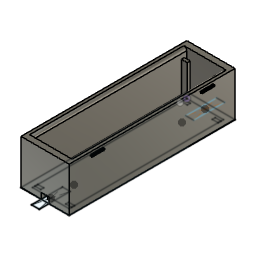
single battery holder and lid 5 (Autodesk Fusion 360 design; units mm, degrees)
Autodesk Fusion 360 part; units mm, degrees
note: some values were not read from the file. Set by a fixed rule: which face or edge a step refers to.
sketch "Sketch1" plane through (0, 0, 0) normal (0, 0, 1) x (1, 0, 0)
  line L0 (0, 0) -> (19, 0)
  line L1 (19, 0) -> (19, -80)
  line L2 (19, -80) -> (0, -80)
  line L3 (0, -80) -> (0, 0)
  line L4 (22, 3) -> (22, -83)
  line L5 (22, -83) -> (-3, -83)
  line L6 (-3, -83) -> (-3, 3)
  line L7 (-3, 3) -> (22, 3)
  line L8 (0, -3.5) -> (0, -1.25)
  line L9 (19, -1.25) -> (16, -1.25)
  line L10 (16, -1.25) -> (16, -2.75)
  line L11 (16, -2.75) -> (19, -2.75)
  line L12 (19, -2.75) -> (19, -1.25)
  line L13 (0, -77.25) -> (3, -77.25)
  line L14 (3, -77.25) -> (3, -78.75)
  line L15 (3, -78.75) -> (0, -78.75)
  line L16 (0, -78.75) -> (0, -77.25)
  line L17 (19, -77.25) -> (16, -77.25)
  line L18 (16, -77.25) -> (16, -78.75)
  line L19 (16, -78.75) -> (19, -78.75)
  line L20 (19, -78.75) -> (19, -77.25)
  line L21 (0, -1.25) -> (3, -1.25)
  line L22 (3, -1.25) -> (3, -2.75)
  line L23 (3, -2.75) -> (0, -2.75)
  line L24 (0, -2.75) -> (0, -1.25)
  line L25 (11.5, -8) -> (7.5, -8)
  line L26 (7.5, -8) -> (7.5, 8)
  line L27 (7.5, 8) -> (11.5, 8)
  line L28 (11.5, 8) -> (11.5, -8)
  line L29 (11.5, -8) -> (7.5, 8) construction
  line L30 (7.5, -8) -> (11.5, 8) construction
  line L31 (11.5, -88) -> (7.5, -88)
  line L32 (7.5, -88) -> (7.5, -72)
  line L33 (7.5, -72) -> (11.5, -72)
  line L34 (11.5, -72) -> (11.5, -88)
  line L35 (11.5, -88) -> (7.5, -72) construction
  line L36 (7.5, -88) -> (11.5, -72) construction
  point P0 (9.5, 0)
  point P1 (9.5, -80)
  point P2 (9.5, -12)
  point P3 (9.5, -68)
  dimension "d1" = 80
  dimension "d2" = 19
  dimension "d3" = -3
  dimension "d5" = 3
  dimension "d6" = 1.5
  dimension "d7" = 3
  dimension "d8" = 1.5
  dimension "d9" = 3
  dimension "d10" = 1.5
  dimension "d11" = 1.5
  dimension "d12" = 3
  dimension "d13" = 1.25
  dimension "d14" = 1.25
  dimension "d15" = 1.25
  dimension "d16" = 1.25
  dimension "d19" = 12
  dimension "d20" = 12
  dimension "d28" = 16
  dimension "d29" = 16
  dimension "d30" = 4
  constraint horizontal L0
  constraint vertical L1
  constraint horizontal L2
  constraint vertical L3
  constraint coincident L0.start L3.end
  constraint vertical L8
  constraint coincident L3 L8.end
  constraint horizontal L9
  constraint vertical L10
  constraint horizontal L11
  constraint vertical L12
  constraint coincident L1 L9.start
  constraint horizontal L13
  constraint vertical L14
  constraint horizontal L15
  constraint vertical L16
  constraint coincident L3 L13.start
  constraint horizontal L17
  constraint vertical L18
  constraint horizontal L19
  constraint vertical L20
  constraint coincident L1 L17.start
  constraint horizontal L21
  constraint vertical L22
  constraint horizontal L23
  constraint vertical L24
  constraint perpendicular L25 L26
  constraint parallel L25 L27
  constraint parallel L26 L28
  constraint horizontal L25
  constraint coincident L29 P0
  constraint coincident L30 P0
  constraint midpoint L0 P0
  constraint perpendicular L31 L32
  constraint parallel L31 L33
  constraint parallel L32 L34
  constraint horizontal L31
  constraint coincident L35 P1
  constraint coincident L36 P1
  constraint midpoint L2 P1
  constraint vertical P1 P3
  constraint vertical P0 P2
  measures "d1" distance of L0.start L2.end
  measures "d2" distance of L0.start L0.end
  measures "d5" distance of L9.start L9.end
  measures "d6" distance of L9.start L11.end
  measures "d7" distance of L13.start L13.end
  measures "d8" distance of L13.start L15.end
  measures "d9" distance of L17.start L17.end
  measures "d10" distance of L17.start L19.end
  measures "d11" distance of L8.end L23.end
  measures "d12" distance of L8.end L21.end
  measures "d13" distance of L0 L21.end
  measures "d14" distance of L0 L9.end
  measures "d15" distance of L2 L14.end
  measures "d16" distance of L2 L18.end
  measures "d19" distance of L0 P2
  measures "d20" distance of L2 P3
  measures "d28" distance of L25.end L26.end
  measures "d29" distance of L31.end L32.end
  measures "d30" distance of L32.end L33.end
extrude "Extrude1" add sketch "Sketch1" along normal blind 3 contours L0 L1 L2 L3 L8 L9 L10 L11 L13 L14 L15 L17 L18 L19 L21 L22 L23 L25 L26 L28 L32 L33 L34 makes body 1
extrude "Extrude1'" add sketch "Sketch1" along normal blind 23 separate body contours L0 L2 L3 L5 L6 L7 L8 L16 L24 L26 L32 | L0 L7 L26 L28 | L0 L1 L2 L4 L5 L7 L12 L20 L28 L34 | L2 L5 L32 L34 makes body 2 in component "single battery holder"
sketch "Sketch1 (2)" plane through (0, 0, 0) normal (0, -1, 0) x (1, 0, 0) in component "single battery holder"
  line L0 (0, 0) -> (19, 0)
  line L1 (19, 0) -> (19, 23)
  line L2 (19, 23) -> (0, 23)
  line L3 (0, 23) -> (0, 0)
  line L4 (-3, 0) -> (22.0074, 23) construction
  line L5 (22.0074, 23) -> (-3, 23) construction
  line L6 (-3, 23) -> (22, 0) construction
  circle A0 centre (9.5037, 11.5) radius 9.5
  dimension "d23" = 19
  constraint perpendicular L3 L5
  constraint midpoint L4 A0.centre
  measures "d23" diameter of A0
extrude "Extrude2" cut sketch "Sketch1 (2)" along normal blind 80 contours L1 A0 | L1 A0 bodies 2 in component "single battery holder"
extrude "Extrude3" add sketch "Sketch1" along normal blind 19 contours L3 L8 L21 L22 L23 L24 | L1 L9 L10 L11 L12 | L3 L13 L14 L15 L16 | L1 L17 L18 L19 L20 bodies 2 in component "single battery holder"
fillet "Fillet1" radius 1.5 2 edges at (0, -40, 23) (19, -40, 23) on bodies 2 in component "single battery holder"
hole "Hole1" at (9.5, -17, 3) direction (0, 0, -1) diameter 3 depth 4 tip angle 180 countersink diameter 4.5 countersink angle 90 bodies 1
hole "Hole2" at (9.5, -63, 3) direction (0, 0, -1) diameter 3 depth 4 tip angle 118 countersink diameter 4.5 countersink angle 90 bodies 1
extrude "Extrude6" cut sketch "Sketch1" along normal blind 3 contours L0 L7 L26 L28 | L2 L5 L32 L34 bodies 2 in component "single battery holder"
sketch "Sketch2" plane through (-3, 0, 0) normal (-1, 0, 0) x (0, -1, 0) in component "single battery holder"
  line L0 (-3, 0) -> (83, 0)
  line L1 (83, 0) -> (83, 23)
  line L2 (83, 23) -> (-3, 23)
  line L3 (-3, 23) -> (-3, 0)
  line L4 (-3, 23) -> (83, 0) construction
  line L5 (-3, 0) -> (83, 23) construction
  line L6 (35, 13) -> (45, 10) construction
  line L7 (45, 13) -> (35, 10) construction
  point P0 (40, 11.5)
  constraint coincident L2.end L3.start
  constraint coincident L0.end L1.start
  constraint coincident L0.start L3.end
  constraint coincident L1.end L2.start
  constraint coincident L6 P0
  constraint coincident L7 P0
  constraint midpoint L5 P0
combine "Combine1" operation add target body 2 tool bodies 1 in component "single battery holder"
ref_plane "WorkPlane1" through (9.5, -83.25, 11.5) normal (0, -1, 0) x (1, 0, 0) in component "Lid4"
sketch "Sketch1 (3)" plane through (9.5, -83.25, 11.5) normal (0, -1, 0) x (1, 0, 0) in component "Lid4"
  line L0 (2, -8.5) -> (2, -11.5)
  line L1 (2, -11.5) -> (12.5, -11.5)
  line L2 (12.5, -11.5) -> (12.5, 11.5)
  line L3 (12.5, 11.5) -> (-12.5, 11.5)
  line L4 (-12.5, 11.5) -> (-12.5, -11.5)
  line L5 (-12.5, -11.5) -> (-2, -11.5)
  line L6 (-2, -11.5) -> (-2, -8.5)
  line L7 (-2, -8.5) -> (2, -8.5)
  line L8 (-13, 7.9743) -> (-15, 7.9743)
  line L9 (-15, 7.9743) -> (-15, 13.501)
  line L10 (-15, 13.501) -> (15, 13.501)
  line L11 (15, 13.501) -> (15, 7.9743)
  line L12 (15, 7.9743) -> (13, 7.9743)
  line L13 (13, 7.9743) -> (13, 11.501)
  line L14 (13, 11.501) -> (-13, 11.501)
  line L15 (-13, 11.501) -> (-13, 7.9743)
  line L16 (0, 11.5) -> (0, 21.153) construction
  line L17 (-12.5, -11.5) -> (-12.5, 11.5)
  line L18 (12.5074, 11.5) -> (-12.5, 11.5)
  dimension "d157" = 0.5
  dimension "d158" = 2
  dimension "d159" = 0.001
  dimension "d160" = 2
  constraint perpendicular L4 L8
  constraint perpendicular L8 L9
  constraint perpendicular L4 L10
  constraint perpendicular L10 L11
  constraint perpendicular L11 L12
  constraint perpendicular L12 L13
  constraint perpendicular L11 L14
  constraint perpendicular L8 L15
  constraint midpoint L3 L16.start
  constraint perpendicular L3 L16
  constraint symmetric L8.start L12.end L16
  constraint symmetric L8.end L11.end L16
  measures "d157" distance of L8.start L17
  measures "d158" distance of L8.start L8.end
  measures "d159" distance of L14 L18
  measures "d160" distance of L10 L14
extrude "Extrude1''" add sketch "Sketch1 (3)" along normal blind 0.35 and the other way blind 86.75 separate body contours L3 L8 L9 L10 L11 L12 L13 L14 L15 L18 makes body 3 in component "Lid4"
sketch "Sketch2 (2)" plane through (24.5, 0, 0) normal (1, 0, 0) x (0, 1, 0) in component "Lid4"
  line L0 (3.5, 25.001) -> (-83.6, 25.001)
  line L1 (-83.6, 25.001) -> (-83.6, 19.4743)
  line L2 (-83.6, 19.4743) -> (3.5, 19.4743)
  line L3 (3.5, 19.4743) -> (3.5, 25.001)
  line L4 (-83, 0) -> (3, 0)
  line L5 (3, 0) -> (3, 23)
  line L6 (3, 23) -> (-83, 23)
  line L7 (-83, 23) -> (-83, 0)
  line L8 (-83.6, 23) -> (3.5, 23) construction
  line L9 (-83.6, 23) -> (3.5, 23) construction
  line L10 (3.5, 23) -> (3.5, 19.4743) construction
  line L11 (3.5, 19.4743) -> (-83.6, 19.4743) construction
  line L12 (-83.6, 19.4743) -> (-83.6, 23) construction
  line L13 (-71.6, 20.4871) -> (-65.6, 20.4871)
  arc A0 (-65.6, 20.4871) -> (-65.6, 21.9871) centre (-65.6, 21.2371) ccw
  line L14 (-65.6, 21.9871) -> (-71.6, 21.9871)
  arc A1 (-71.6, 21.9871) -> (-71.6, 20.4871) centre (-71.6, 21.2371) ccw
  line L15 (-71.6, 21.2371) -> (-65.6, 21.2371) construction
  line L16 (-43.05, 20.4871) -> (-37.05, 20.4871)
  line L17 (-43.05, 21.2371) -> (-37.05, 21.2371) construction
  arc A2 (-37.05, 20.4871) -> (-37.05, 21.9871) centre (-37.05, 21.2371) ccw
  line L18 (-37.05, 21.9871) -> (-43.05, 21.9871)
  arc A3 (-43.05, 21.9871) -> (-43.05, 20.4871) centre (-43.05, 21.2371) ccw
  line L19 (-8.5, 21.9871) -> (-14.5, 21.9871)
  line L20 (-14.5, 20.4871) -> (-8.5, 20.4871)
  arc A4 (-14.5, 21.9871) -> (-14.5, 20.4871) centre (-14.5, 21.2371) ccw
  arc A5 (-8.5, 20.4871) -> (-8.5, 21.9871) centre (-8.5, 21.2371) ccw
  line L21 (-14.5, 21.2371) -> (-8.5, 21.2371) construction
  point P0 (-68.6, 21.2371)
  point P1 (-40.05, 21.2371)
  point P2 (-11.5, 21.2371)
  point P3 (-68.6, 21.2371)
  dimension "d165" = 3.5257
  dimension "d166" = 1.7629
  dimension "d168" = 15
  dimension "d169" = 15
  dimension "d170" = 43.55
  dimension "d171" = 3
  dimension "d172" = 1.5
  dimension "d173" = 1.5
  dimension "d174" = 1.5
  constraint coincident L1 L8.start
  constraint coincident L3 L8.end
  constraint perpendicular L5 L8
  constraint horizontal L9
  constraint vertical L10
  constraint horizontal L11
  constraint vertical L12
  constraint coincident L2.end L3.start
  constraint horizontal P3 P1
  constraint horizontal P1 P2
  constraint tangent L13 A0
  constraint tangent A0 L14
  constraint parallel L13 L14
  constraint tangent L14 A1
  constraint tangent L13 A1
  constraint parallel L8 L15
  constraint coincident P3 P0
  constraint midpoint L15 P3
  constraint tangent L16 A2
  constraint tangent A2 L18
  constraint parallel L16 L18
  constraint tangent L18 A3
  constraint tangent L16 A3
  constraint tangent L20 A5
  constraint tangent L19 A5
  constraint parallel L19 L20
  constraint tangent L19 A4
  constraint tangent L20 A4
  measures "d165" distance of L1.end L8.start
  measures "d166" distance of L8 P3
  measures "d168" distance of L12 P3
  measures "d169" distance of L3 P2
  measures "d170" distance of L10 P1
  measures "d171" distance of A0.centre P3
  measures "d172" diameter of A0
  measures "d173" diameter of A2
  measures "d174" diameter of A5
extrude "Extrude2'" cut sketch "Sketch2 (2)" along normal blind -3 and the other way blind 1 contours L13 A0 L14 A1 | L19 L20 A4 A5 bodies 3 in component "Lid4"
sketch "Sketch6" plane through (22, 0, 0) normal (1, 0, 0) x (0, 1, 0) in component "single battery holder"
  line L0 (-83, 0) -> (3, 0)
  line L1 (3, 0) -> (3, 23)
  line L2 (3, 23) -> (-83, 23)
  line L3 (-83, 23) -> (-83, 0)
  arc A0 (-8.5, 20.4871) -> (-8.5, 21.9871) centre (-8.5, 21.2371) ccw construction
  line L4 (-8.5, 20.4871) -> (-14.5, 20.4871) construction
  arc A1 (-14.5, 21.9871) -> (-14.5, 20.4871) centre (-14.5, 21.2371) ccw construction
  line L5 (-14.5, 21.9871) -> (-8.5, 21.9871) construction
  arc A2 (-71.6, 21.9871) -> (-71.6, 20.4871) centre (-71.6, 21.2371) ccw construction
  line L6 (-71.6, 21.9871) -> (-65.6, 21.9871) construction
  arc A3 (-65.6, 20.4871) -> (-65.6, 21.9871) centre (-65.6, 21.2371) ccw construction
  line L7 (-65.6, 20.4871) -> (-71.6, 20.4871) construction
  line L8 (-71.6, 21.2371) -> (-65.6, 21.2371) construction
  line L9 (-71.6, 20.6871) -> (-65.6, 20.6871)
  arc A4 (-65.6, 20.6871) -> (-65.6, 21.7871) centre (-65.6, 21.2371) ccw
  line L10 (-65.6, 21.7871) -> (-71.6, 21.7871)
  arc A5 (-71.6, 21.7871) -> (-71.6, 20.6871) centre (-71.6, 21.2371) ccw
  line L11 (-71.6, 21.2371) -> (-65.6, 21.2371) construction
  line L12 (-8.5, 21.2371) -> (-14.5, 21.2371) construction
  line L13 (-14.5, 20.6871) -> (-8.5, 20.6871)
  arc A6 (-8.5, 20.6871) -> (-8.5, 21.7871) centre (-8.5, 21.2371) ccw
  line L14 (-8.5, 21.7871) -> (-14.5, 21.7871)
  arc A7 (-14.5, 21.7871) -> (-14.5, 20.6871) centre (-14.5, 21.2371) ccw
  line L15 (-14.5, 21.2371) -> (-8.5, 21.2371) construction
  point P0 (-68.6, 21.2371)
  point P1 (-11.5, 21.2371)
  dimension "d179" = 1.1
  dimension "d180" = 1.1
  constraint coincident A2.centre L8.start
  constraint coincident A3.centre L8.end
  constraint tangent L9 A4
  constraint tangent A4 L10
  constraint parallel L9 L10
  constraint tangent L10 A5
  constraint tangent L9 A5
  constraint parallel L8 L11
  constraint midpoint L8 P0
  constraint midpoint L11 P0
  constraint coincident A0.centre L12.start
  constraint coincident A1.centre L12.end
  constraint tangent L13 A6
  constraint tangent A6 L14
  constraint parallel L13 L14
  constraint tangent L14 A7
  constraint tangent L13 A7
  constraint parallel L12 L15
  constraint midpoint L12 P1
  constraint midpoint L15 P1
  measures "d179" diameter of A4
  measures "d180" diameter of A6
extrude "Extrude11" add sketch "Sketch6" along normal blind 0.75 contours L9 A4 L10 A5 | L13 A6 L14 A7 bodies 2 in component "single battery holder"
fillet "Fillet5" radius 0.25 2 faces at (22.75, -10.5, 21.0538) (22.75, -67.6, 21.0538) on bodies 2 in component "single battery holder"
sketch "Sketch3" plane through (-5.5, 0, 0) normal (-1, 0, 0) x (0, -1, 0) in component "Lid4"
  line L0 (-3.5, 19.4743) -> (83.6, 19.4743)
  line L1 (83.6, 19.4743) -> (83.6, 25.001)
  line L2 (83.6, 25.001) -> (-3.5, 25.001)
  line L3 (-3.5, 25.001) -> (-3.5, 19.4743)
  line L4 (43.05, 21.2371) -> (37.05, 21.2371)
  line L5 (37.05, 21.9871) -> (43.05, 21.9871)
  line L6 (43.05, 20.4871) -> (37.05, 20.4871)
  arc A0 (43.05, 20.4871) -> (43.05, 21.9871) centre (43.05, 21.2371) ccw
  arc A1 (37.05, 21.9871) -> (37.05, 20.4871) centre (37.05, 21.2371) ccw
  line L7 (37.05, 20.4871) -> (43.05, 20.4871)
  arc A2 (43.05, 20.4871) -> (43.05, 21.9871) centre (43.05, 21.2371) ccw
  line L8 (43.05, 21.9871) -> (37.05, 21.9871)
  arc A3 (37.05, 21.9871) -> (37.05, 20.4871) centre (37.05, 21.2371) ccw
  line L9 (37.05, 21.2371) -> (43.05, 21.2371) construction
  point P0 (40.05, 21.2371)
  constraint tangent L7 A2
  constraint tangent A2 L8
  constraint parallel L7 L8
  constraint tangent L8 A3
  constraint tangent L7 A3
  constraint coincident L4.start A0.centre
  constraint parallel L4 L9
  constraint midpoint L4 P0
  constraint midpoint L9 P0
extrude "Extrude3'" cut sketch "Sketch3" along normal blind -1 and the other way blind 3 contours L5 L6 A0 A1 L7 A2 L8 A3 bodies 3 in component "Lid4"
sketch "Sketch7" plane through (-3, 0, 0) normal (-1, 0, 0) x (0, -1, 0) in component "single battery holder"
  line L0 (43.05, 21.2371) -> (37.05, 21.2371)
  line L1 (37.05, 21.9871) -> (43.05, 21.9871)
  line L2 (43.05, 20.4871) -> (37.05, 20.4871)
  arc A0 (37.05, 21.9871) -> (37.05, 20.4871) centre (37.05, 21.2371) ccw
  arc A1 (43.05, 20.4871) -> (43.05, 21.9871) centre (43.05, 21.2371) ccw
  line L3 (37.05, 20.6871) -> (43.05, 20.6871)
  arc A2 (43.05, 20.6871) -> (43.05, 21.7871) centre (43.05, 21.2371) ccw
  line L4 (43.05, 21.7871) -> (37.05, 21.7871)
  arc A3 (37.05, 21.7871) -> (37.05, 20.6871) centre (37.05, 21.2371) ccw
  line L5 (37.05, 21.2371) -> (43.05, 21.2371) construction
  point P0 (40.05, 21.2371)
  dimension "d188" = 1.1
  constraint tangent L3 A2
  constraint tangent A2 L4
  constraint parallel L3 L4
  constraint tangent L4 A3
  constraint tangent L3 A3
  constraint coincident L0.start A1.centre
  constraint parallel L0 L5
  constraint midpoint L0 P0
  constraint midpoint L5 P0
  measures "d188" diameter of A2
extrude "Extrude12" add sketch "Sketch7" along normal blind 0.75 contours L3 A2 L4 A3 bodies 2 in component "single battery holder"
fillet "Fillet6" radius 0.25 1 faces at (-3.75, -41.05, 21.0538) on bodies 2 in component "single battery holder"
sketch "Sketch4" plane through (0, -83.6, 0) normal (0, -1, 0) x (1, 0, 0) in component "Lid4"
  line L0 (-3.5, 23.001) -> (22.5, 23.001)
  line L1 (22.5, 23.001) -> (22.5, 19.4743)
  line L2 (22.5, 19.4743) -> (24.5, 19.4743)
  line L3 (24.5, 19.4743) -> (24.5, 25.001)
  line L4 (24.5, 25.001) -> (-5.5, 25.001)
  line L5 (-5.5, 25.001) -> (-5.5, 19.4743)
  line L6 (-5.5, 19.4743) -> (-3.5, 19.4743)
  line L7 (-3.5, 19.4743) -> (-3.5, 23.001)
  line L8 (-5.5, 25.001) -> (24.5, 25.001)
  line L9 (24.5, 25.001) -> (24.5, 19.4743)
  line L10 (24.5, 19.4743) -> (-5.5, 19.4743)
  line L11 (-5.5, 19.4743) -> (-5.5, 25.001)
  constraint horizontal L8
  constraint vertical L9
  constraint horizontal L10
  constraint vertical L11
  constraint coincident L2.end L3.start
  constraint coincident L4.end L5.start
sketch "Sketch5" plane through (0, 3.5, 0) normal (0, 1, 0) x (-1, 0, 0) in component "Lid4"
  line L0 (-22.5, 23.001) -> (3.5, 23.001)
  line L1 (3.5, 23.001) -> (3.5, 19.4743)
  line L2 (3.5, 19.4743) -> (5.5, 19.4743)
  line L3 (5.5, 19.4743) -> (5.5, 25.001)
  line L4 (5.5, 25.001) -> (-24.5, 25.001)
  line L5 (-24.5, 25.001) -> (-24.5, 19.4743)
  line L6 (-24.5, 19.4743) -> (-22.5, 19.4743)
  line L7 (-22.5, 19.4743) -> (-22.5, 23.001)
  line L8 (-24.5, 25.001) -> (5.5, 25.001)
  line L9 (5.5, 25.001) -> (5.5, 19.4743)
  line L10 (5.5, 19.4743) -> (-24.5, 19.4743)
  line L11 (-24.5, 19.4743) -> (-24.5, 25.001)
  constraint horizontal L8
  constraint vertical L9
  constraint horizontal L10
  constraint vertical L11
  constraint coincident L2.end L3.start
  constraint coincident L4.end L5.start
fillet "Fillet2" radius 0.5 16 faces at (4.5, -83.3667, 25.001) (4.5, -54.3333, 25.001) (24.5, -83.3667, 23.1588) (24.5, -54.3333, 23.1588) (23.8333, -83.3667, 19.4743) (23.8333, -54.3333, 19.4743) (-4.1667, -83.3667, 19.4743) (-4.1667, -54.3333, 19.4743) (-5.5, -83.3667, 21.3165) (-5.5, -54.3333, 21.3165) (13.6667, 3.5, 24.3343) (13.6667, -83.6, 24.3343) (22.5, -83.3667, 20.6499) (22.5, -0.25, 21.2375) (-3.5, -83.3667, 21.8254) (-3.5, -9.7667, 21.2375) on bodies 3 in component "Lid4"
sketch "Sketch6 (2)" plane through (-5.5, 0, 0) normal (-1, 0, 0) x (0, -1, 0) in component "Lid4"
  line L0 (-3, 24.501) -> (-3, 19.9743)
  line L1 (83.1, 19.9743) -> (83.1, 24.501)
  line L2 (83.1, 24.501) -> (-3, 24.501)
  line L3 (37.1, 20.4743) -> (43, 20.4743)
  arc A0 (43, 20.4743) -> (43, 22) centre (43, 21.2371) ccw
  line L4 (43, 22) -> (37.1, 22)
  arc A1 (37.1, 22) -> (37.1, 20.4743) centre (37.1, 21.2371) ccw
  line L5 (37.1, 21.2371) -> (43, 21.2371) construction
  line L6 (-3, 19.9743) -> (83.1, 19.9743)
  point P0 (40.05, 21.2371)
  point P1 (40.05, 21.2371)
  constraint tangent L3 A0
  constraint tangent A0 L4
  constraint parallel L3 L4
  constraint tangent L4 A1
  constraint tangent L3 A1
  constraint coincident P1 P0
  constraint midpoint L5 P1
extrude "Extrude6'" add sketch "Sketch6 (2)" along normal blind 1.5 contours L3 A0 L4 A1 bodies 3 in component "Lid4"
fillet "Fillet3" radius 0.25 1 faces at (-7, -41.0333, 20.9829) on bodies 3 in component "Lid4"
fillet "Fillet4" [suppressed] in component "single battery holder"
component "single battery holder" placed x (1, 0, 0) y (0, 1, 0) z (0, 0, 1) at (0, 0, 0)
component "Lid4" placed x (1, 0, 0) y (0, 1, 0) z (0, 0, 1) at (0, 0, 0)
equation "d14 = d13"
equation "d15 = d13"
equation "d16 = d13"
equation "d20 = d19"
equation "d166 = d165 / 2"
equation "d169 = d168"
equation "d170 = ( 87.1 / 2 ) * 1 mm"
